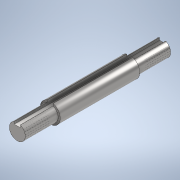
# Autodesk Inventor part: HornGearShaft
Saved by Autodesk Inventor 2022 (Build 260153070, 153G)
## iProperties
Created: 2021-06-02
Part Number: HornGearShaft
Material: Stainless Steel
Document SubType Name: Modeling
Designer: Eric
Density: 8 g/cm^3
Appearance: Semi-Polished
Author: Eric
Autodesk Inventor part; units mm, degrees
ref_plane "YZ Plane" through (0, 0, 0) normal (1, 0, 0) x (0, 1, 0)
ref_plane "XZ Plane" through (0, 0, 0) normal (0, 1, 0) x (-1, 0, 0)
ref_plane "XY Plane" through (0, 0, 0) normal (0, 0, 1) x (1, 0, 0)
sketch "Sketch1" plane through (0, 0, 0) normal (0, 0, 1) x (1, 0, 0)
  circle A0 centre (0, 0) radius 5
  dimension "d0" = 10
  constraints: 1 centre point, 1 coincident
  measures "d0" diameter of A0
extrude "Extrusion1" add sketch "Sketch1" along normal mid plane 40
sketch "Sketch2" plane through (0, 0, 20) normal (0, 0, 1) x (1, 0, 0)
  circle A0 centre (0, 0) radius 4
  line L0 (-2.6458, 3) -> (2.6458, 3)
  line L1 (1.5, 2.5) -> (1.5, 5.5)
  line L2 (1.5, 5.5) -> (-1.5, 5.5)
  line L3 (-1.5, 5.5) -> (-1.5, 2.5)
  line L4 (-1.5, 2.5) -> (1.5, 2.5)
  line L5 (1.5, 2.5) -> (-1.5, 5.5) construction
  line L6 (1.5, 5.5) -> (-1.5, 2.5) construction
  line L7 (0, -7.1) -> (0, 7.6) projected
  point P0 (0, 4)
  point P1 (0, 4)
  point P2 (-1.5, 3.7081)
  point P3 (1.5, 3.7081)
  dimension "d3" = 8
  dimension "d4" = 3
  dimension "d11" = 3
  dimension "d12" = 3
  constraints: 14 end point, 3 midpoint, 3 point on circle, 2 parallel, 1 centre point, 1 coincident, 1 horizontal, 1 perpendicular, 1 point on line, 1 vertical
  measures "d3" diameter of A0
  measures "d4" distance from line of point (0, 0) L0
  measures "d11" distance of L1.start L1.end
  measures "d12" distance of L1.end L2.end
extrude "Extrusion2" add sketch "Sketch2" along normal blind 16.5 contours A0 L7 L4 L1 L0 | L0 L1 A0 | A0 L0 L3 L4 L7 | L1 L0 L7 A0 | L1 L4 L7 L0 | A0 L3 L0 | L4 L3 L0 L7 | L7 L0 L3 A0
thread "Thread1" size "M8x1.25" class "6g" standard "ANSI Metric M Profile" length 12.5 offset 4
mirror "Mirror2" about plane through (0, 0, 0) normal (0, 0, 1) of "Extrusion2"
thread "Thread2" size "M8x1.25" class "6g" standard "ANSI Metric M Profile" length 12.5 offset 4
extrude "Extrusion3" cut sketch "Sketch2" along normal through all both and the other way through all contours L1 L0 L7 A0 | A0 L7 L2 L1 | L1 L4 L7 L0 | L4 L3 L0 L7 | L7 L0 L3 A0 | A0 L3 L2 L7
body "Solid1"
